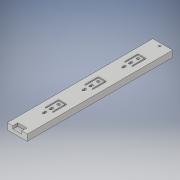
# Autodesk Inventor part: drawer rails
Saved by Autodesk Inventor 2017 (Build 210142000, 142)
## iProperties
Created: 2018-12-20
Part Number: drawer rails
Material: Generic
Document SubType Name: Modeling
Designer: 309524
Density: 1 g/cm^3
Appearance: Default
Author: 309524
Autodesk Inventor part; units mm, degrees
ref_plane "YZ Plane" through (0, 0, 0) normal (1, 0, 0) x (0, 1, 0)
ref_plane "XZ Plane" through (0, 0, 0) normal (0, 1, 0) x (-1, 0, 0)
ref_plane "XY Plane" through (0, 0, 0) normal (0, 0, 1) x (1, 0, 0)
sketch "Sketch1" plane through (0, 0, 0) normal (0, 1, 0) x (-1, 0, 0)
  line L0 (-23.9141, 174.625) -> (23.9141, 174.625)
  line L1 (23.9141, 174.625) -> (23.9141, -174.625)
  line L2 (23.9141, -174.625) -> (-23.9141, -174.625)
  line L3 (-23.9141, -174.625) -> (-23.9141, 174.625)
  line L4 (-23.9141, 174.625) -> (23.9141, -174.625) construction
  line L5 (23.9141, 174.625) -> (-23.9141, -174.625) construction
  point P0 (0, 0)
  dimension "d0" = 47.8282
  dimension "d1" = 349.25
  constraints: 12 end point, 2 midpoint, 2 parallel, 1 horizontal, 1 perpendicular
  measures "d0" distance of L1.end L2.end
  measures "d1" distance of L0.end L1.end
extrude "Extrusion1" add sketch "Sketch1" along normal blind 15.0622
sketch "Sketch2" plane through (0, 15.0622, 0) normal (0, 1, 0) x (1, 0, 0)
  line L0 (-10.6299, -174.625) -> (10.6426, -174.625)
  line L1 (10.6426, -174.625) -> (10.6426, -162.4584)
  line L2 (10.6426, -162.4584) -> (-10.6299, -162.4584)
  line L3 (-10.6299, -162.4584) -> (-10.6299, -174.625)
  line L4 (-23.9141, -174.625) -> (23.9141, -174.625) projected
  line L5 (-23.9141, 174.625) -> (-23.9141, -174.625) projected
  point P0 (0, 0)
  point P1 (0, -132.6268)
  dimension "d4" = 21.2725
  dimension "d5" = 12.1666
  dimension "d6" = 13.2842
  dimension "d7" = 23.9141
  constraints: 8 end point, 2 parallel, 1 collinear, 1 horizontal, 1 perpendicular
  measures "d4" distance of L2.end L1.end
  measures "d5" distance of L0.end L1.end
  measures "d6" distance between parallel lines of L3 L5
  measures "d7" distance from line of point (0, -132.627) L5
extrude "Extrusion2" cut sketch "Sketch2" against normal blind 6.858
sketch "Sketch3" plane through (0, 15.0622, 0) normal (0, 1, 0) x (1, 0, 0)
  circle A0 centre (0, -111.252) radius 2.1336
  line L0 (-10.6299, -162.4584) -> (10.6426, -162.4584) projected
  circle A1 centre (0.0065, -106.299) radius 2.1336
  line L1 (-2.1271, -106.2962) -> (-2.1336, -111.2492)
  line L2 (2.1401, -106.3018) -> (2.1336, -111.2548)
  line L3 (0.0064, -93.8649) -> (0.0064, -74.1654) construction
  circle A2 centre (0, -94.9706) radius 2.1336
  circle A3 centre (0.0065, -90.0176) radius 2.1336
  line L4 (-2.1271, -90.0148) -> (-2.1336, -94.9678)
  line L5 (2.1401, -90.0204) -> (2.1336, -94.9734)
  circle A4 centre (0, -16.002) radius 2.1336
  circle A5 centre (0.0065, -11.049) radius 2.1336
  line L6 (-2.1271, -11.0462) -> (-2.1336, -15.9992)
  line L7 (2.1401, -11.0518) -> (2.1336, -16.0048)
  circle A6 centre (0, 0.2794) radius 2.1336
  circle A7 centre (0.0065, 5.2324) radius 2.1336
  line L8 (-2.1271, 5.2352) -> (-2.1336, 0.2822)
  line L9 (2.1401, 5.2296) -> (2.1336, 0.2766)
  circle A8 centre (0, 79.248) radius 2.1336
  circle A9 centre (0.0065, 84.201) radius 2.1336
  line L10 (-2.1271, 84.2038) -> (-2.1336, 79.2508)
  line L11 (2.1401, 84.1982) -> (2.1336, 79.2452)
  circle A10 centre (0, 95.5294) radius 2.1336
  circle A11 centre (0.0065, 100.4824) radius 2.1336
  line L12 (-2.1271, 100.4852) -> (-2.1336, 95.5322)
  line L13 (2.1401, 100.4796) -> (2.1336, 95.5266)
  point P0 (0, 0)
  point P1 (0.0064, 1.3851)
  point P2 (0.0064, 96.6351)
  dimension "d10" = 4.2672
  dimension "d11" = 51.2064
  dimension "d12" = 4.2672
  dimension "d13" = 9.2202
  dimension "d18" = 16.2814
  dimension "d34" = 95.25
  constraints: 26 end point, 24 point on circle, 12 centre point, 4 tangent, 3 vertical, 52 other
  measures "d10" diameter of A0
  measures "d11" distance from line of L0 A0.centre
  measures "d12" diameter of A1
  measures "d18" distance of A0.centre A2.centre
  measures "d34" distance of A0.centre A4.centre
sketch "Sketch4" plane through (0, 15.0622, 0) normal (0, 1, 0) x (1, 0, 0)
  line L0 (-9.9568, -97.1042) -> (-9.9568, -65.3542)
  line L1 (-9.9568, -65.3542) -> (9.9568, -65.3542)
  line L2 (9.9568, -65.3542) -> (9.9568, -97.1042)
  arc A0 (-2.1336, -111.2492) -> (2.1336, -111.2548) centre (0, -111.252) ccw construction
  line L3 (-7.4168, -97.1042) -> (-7.4168, -67.8942)
  line L4 (-7.4168, -67.8942) -> (7.4168, -67.8942)
  line L5 (7.4168, -67.8942) -> (7.4168, -97.2756)
  line L6 (-16.8514, -97.1042) -> (16.8246, -97.1042) construction
  arc A1 (-2.1336, -94.9678) -> (2.1336, -94.9734) centre (0, -94.9706) ccw construction
  arc A2 (-9.9568, -97.1042) -> (-7.4168, -97.1042) centre (-8.6868, -97.1042) ccw
  arc A3 (7.4168, -97.2756) -> (9.9568, -97.1042) centre (8.6926, -97.2756) ccw
  circle A4 centre (0, -75.2158) radius 3.175
  line L7 (0, 24.1867) -> (0, 36.4789) construction
  arc A5 (-9.9568, -1.8542) -> (-7.4168, -1.8542) centre (-8.6868, -1.8542) ccw
  arc A6 (7.4168, -2.0256) -> (9.9568, -1.8542) centre (8.6926, -2.0256) ccw
  circle A7 centre (0, 20.0342) radius 3.175
  line L8 (-7.4168, -1.8542) -> (-7.4168, 27.3558)
  line L9 (7.4168, 27.3558) -> (7.4168, -2.0256)
  line L10 (-7.4168, 27.3558) -> (7.4168, 27.3558)
  line L11 (-9.9568, 29.8958) -> (9.9568, 29.8958)
  line L12 (9.9568, 29.8958) -> (9.9568, -1.8542)
  line L13 (-9.9568, -1.8542) -> (-9.9568, 29.8958)
  arc A8 (-9.9568, 93.3958) -> (-7.4168, 93.3958) centre (-8.6868, 93.3958) ccw
  arc A9 (7.4168, 93.2244) -> (9.9568, 93.3958) centre (8.6926, 93.2244) ccw
  circle A10 centre (0, 115.2842) radius 3.175
  line L14 (-7.4168, 93.3958) -> (-7.4168, 122.6058)
  line L15 (7.4168, 122.6058) -> (7.4168, 93.2244)
  line L16 (-7.4168, 122.6058) -> (7.4168, 122.6058)
  line L17 (-9.9568, 125.1458) -> (9.9568, 125.1458)
  line L18 (9.9568, 125.1458) -> (9.9568, 93.3958)
  line L19 (-9.9568, 93.3958) -> (-9.9568, 125.1458)
  point P0 (0, 0)
  point P1 (16.8246, -1.8542)
  point P2 (16.8246, 93.3958)
  dimension "d25" = 31.75
  dimension "d26" = 19.9136
  dimension "d28" = 9.9568
  dimension "d29" = 2.54
  dimension "d30" = 0
  dimension "d31" = 6.35
  dimension "d41" = 95.25
  constraints: 40 end point, 12 point on circle, 9 centre point, 4 perpendicular, 3 tangent, 3 vertical, 1 horizontal, 44 other
  measures "d25" distance of L1.end L2.end
  measures "d26" distance of L0.end L1.end
  measures "d28" distance from line of A0.centre L2
  measures "d29" distance between parallel lines of L0 L3
  measures "d30" distance from line of L6 L2.end
  measures "d31" diameter of A4
  measures "d41" distance of L0.start L13.start
extrude "Extrusion5" cut sketch "Sketch4" against normal blind 6.858
extrude "Extrusion6" cut sketch "Sketch3" against normal blind 6.858
sketch "Sketch5" plane through (0, 15.0622, 0) normal (0, 1, 0) x (1, 0, 0)
  circle A0 centre (0, 167.3174) radius 2.3546
  line L0 (23.9141, 174.625) -> (-23.9141, 174.625) projected
  point P0 (0, 0)
  dimension "d50" = 4.7092
  dimension "d51" = 4.953
  constraints: 1 centre point
  measures "d50" diameter of A0
  measures "d51" distance edge to line of A0 L0
extrude "Extrusion7" cut sketch "Sketch5" against normal blind 6.858
sketch "Sketch6" plane through (0, 0, 0) normal (0, -1, 0) x (1, 0, 0)
  circle A0 centre (0, 144.0685) radius 2.159
  circle A1 centre (0, 139.1358) radius 2.159
  line L0 (2.159, 144.0685) -> (2.159, 139.1358)
  line L1 (-2.159, 144.0685) -> (-2.159, 139.1358)
  line L2 (2.4765, 127.6296) -> (-2.4765, 127.6296)
  circle A2 centre (2.4765, 125.4706) radius 2.159
  circle A3 centre (-2.4765, 125.4706) radius 2.159
  line L3 (-0.0635, 119.2045) -> (-0.0635, 135.9892) construction
  line L4 (23.9141, -174.625) -> (23.9141, 174.625) projected
  line L5 (2.4765, 123.3116) -> (-2.4765, 123.3116)
  line L6 (-23.9141, 174.625) -> (-23.9141, -174.625) projected
  circle A4 centre (0, 116.0726) radius 2.159
  line L7 (0, 93.2461) -> (0, 84.503) construction
  line L8 (2.4765, -35.4384) -> (-2.4765, -35.4384)
  circle A5 centre (2.4765, -33.2794) radius 2.159
  circle A6 centre (-2.4765, -33.2794) radius 2.159
  circle A7 centre (0, -19.6142) radius 2.159
  circle A8 centre (0, -42.6774) radius 2.159
  line L9 (2.159, -14.6815) -> (2.159, -19.6142)
  line L10 (-2.159, -14.6815) -> (-2.159, -19.6142)
  line L11 (-0.0635, -39.5455) -> (-0.0635, -22.7608) construction
  line L12 (2.4765, -31.1204) -> (-2.4765, -31.1204)
  circle A9 centre (0, -14.6815) radius 2.159
  line L13 (0, -44.8364) -> (0, -108.3364) construction
  point P0 (0, 0)
  dimension "d54" = 4.318
  dimension "d55" = 4.318
  dimension "d56" = 9.2507
  dimension "d61" = 9.3472
  dimension "d62" = 4.318
  dimension "d63" = 4.318
  dimension "d64" = 9.271
  dimension "d65" = 19.2786
  dimension "d66" = 23.9141
  dimension "d67" = 4.318
  dimension "d68" = 5.08
  dimension "d71" = 158.75
  dimension "d76" = 63.5
  constraints: 24 end point, 16 point on circle, 9 centre point, 7 tangent, 5 vertical, 1 horizontal, 1 line through centre, 1 vertical alignment, 26 other
  measures "d54" diameter of A0
  measures "d55" diameter of A1
  measures "d61" distance edge to line of A1 L2
  measures "d62" diameter of A2
  measures "d63" diameter of A3
  measures "d65" distance edge to line of A2 L4
  measures "d66" distance from line of A1.centre L4
  measures "d67" diameter of A4
  measures "d68" distance edge to line of A4 L5
  measures "d71" distance of A2.centre A5.centre
  measures "d76" distance of L13.start L13.end
sketch "Sketch7" plane through (0, 0, 0) normal (0, -1, 0) x (1, 0, 0)
  circle A0 centre (0, -110.4954) radius 2.159
  line L0 (23.9141, 174.625) -> (-23.9141, 174.625) projected
  line L1 (-23.9141, 174.625) -> (-23.9141, -174.625) projected
  line L2 (-23.9141, -174.625) -> (23.9141, -174.625) projected
  line L3 (23.9141, -174.625) -> (23.9141, 174.625) projected
  circle A1 centre (0, -42.6774) radius 2.159 projected
  circle A2 centre (-0.0001, -115.4484) radius 2.159
  line L4 (2.1589, -115.4484) -> (2.159, -110.4955)
  line L5 (-2.159, -115.423) -> (-2.159, -110.4954)
  circle A3 centre (2.4765, -129.1609) radius 2.159
  circle A4 centre (-2.4757, -129.0705) radius 2.159
  line L6 (2.4765, -131.3199) -> (-2.5149, -131.2291)
  line L7 (2.4739, -127.0019) -> (-2.4361, -126.9118)
  circle A5 centre (0.287, -136.3609) radius 2.159
  line L8 (-23.9141, 174.625) -> (-23.9141, -174.625) projected
  point P0 (0, 0)
  dimension "d79" = 4.318
  dimension "d80" = 63.5
  dimension "d81" = 4.318
  dimension "d82" = 9.271
  dimension "d83" = 4.318
  dimension "d84" = 4.318
  dimension "d85" = 9.271
  dimension "d86" = 21.4376
  dimension "d87" = 9.3472
  dimension "d88" = 4.318
  dimension "d89" = 5.08
  constraints: 8 end point, 8 point on circle, 5 centre point, 4 tangent
  measures "d79" diameter of A0
  measures "d81" diameter of A2
  measures "d83" diameter of A3
  measures "d84" diameter of A4
  measures "d86" distance from line of L3 A3.centre
  measures "d87" distance edge to line of A2 L7
  measures "d88" diameter of A5
  measures "d89" distance from line of L6 A5.centre
extrude "Extrusion10" cut sketch "Sketch6" against normal blind 6.35
extrude "Extrusion11" cut sketch "Sketch7" against normal blind 6.35 contours A0 | L4 A2 L5 A0 | A2 | A3 L6 A4 L7 | A4 | A5
body "Solid1"
